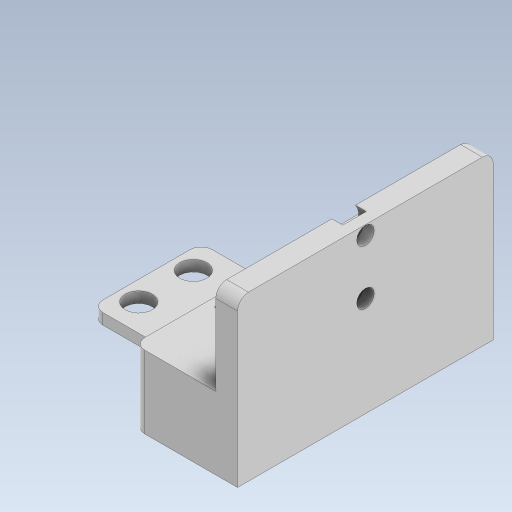
# Autodesk Inventor part: Bracket Servo
Saved by Autodesk Inventor 2023.5 (Build 275446000, 446)
## iProperties
Created: 2025-10-05
Part Number: Bracket Servo
Material: Generic
Document SubType Name: Modeling
Designer: Guntur
Density: 1 g/cm^3
Appearance: Default
Author: Guntur
## iProperties of the stored document Bracket Servo_3DPrint.ipt
Created: 2025-10-05
Part Number: Bracket Servo_3DPrint
Material: Generic
Document SubType Name: Modeling
Designer: Guntur
Density: 1 g/cm^3
Appearance: Default
Author: Guntur
Autodesk Inventor part; units mm, degrees
ref_plane "YZ Plane" through (0, 0, 0) normal (1, 0, 0) x (0, 1, 0)
ref_plane "XZ Plane" through (0, 0, 0) normal (0, 1, 0) x (-1, 0, 0)
ref_plane "XY Plane" through (0, 0, 0) normal (0, 0, 1) x (1, 0, 0)
sketch "Sketch1" plane through (0, 0, 0) normal (0, 1, 0) x (-1, 0, 0)
  line L0 (6, 11.4375) -> (-6, 11.4375)
  line L1 (-6, 11.4375) -> (-6, -11.4375)
  line L2 (-6, -11.4375) -> (6, -11.4375)
  line L3 (6, -11.4375) -> (6, 11.4375)
  line L4 (6, 11.4375) -> (-6, -11.4375) construction
  line L5 (-6, 11.4375) -> (6, -11.4375) construction
  line L6 (6, 16.15) -> (-6, 16.15)
  line L7 (-6, 16.15) -> (-6, -16.15)
  line L8 (-6, -16.15) -> (6, -16.15)
  line L9 (6, -16.15) -> (6, 16.15)
  line L10 (6, 16.15) -> (-6, -16.15) construction
  line L11 (-6, 16.15) -> (6, -16.15) construction
  circle A0 centre (0, -5.4375) radius 2.5
  circle A1 centre (-2.5, 17.225) radius 2.5
  line L12 (7.5, 17.5) -> (-7.5, 17.5)
  line L13 (-7.5, 17.5) -> (-7.5, -17.5)
  line L14 (-7.5, -17.5) -> (7.5, -17.5)
  line L15 (7.5, -17.5) -> (7.5, 17.5)
  line L16 (7.5, 17.5) -> (-7.5, -17.5) construction
  line L17 (-7.5, 17.5) -> (7.5, -17.5) construction
  line L18 (7.5, 17.5) -> (-7.5, 17.5)
  line L19 (-7.5, 17.5) -> (-7.5, 29.3625)
  line L20 (-7.5, 29.3625) -> (7.5, 29.3625)
  line L21 (7.5, 29.3625) -> (7.5, 17.5)
  circle A2 centre (15, 0.9625) radius 2.5
  circle A3 centre (15, 10.9625) radius 2.5
  circle A4 centre (25, 10.9625) radius 2.5
  circle A5 centre (25, 0.9625) radius 2.5
  line L22 (28.6005, 5.9313) -> (28.6005, -4.0687)
  line L23 (28.6005, -4.0687) -> (7.5, -4.0687)
  line L24 (28.6005, 5.9313) -> (28.6005, 15.9313)
  line L25 (28.6005, 15.9313) -> (7.5, 15.9313)
  line L26 (-7.5, -17.5) -> (-11.5, -17.5)
  line L27 (-11.5, -17.5) -> (-11.5, 29.3625)
  line L28 (-11.5, 29.3625) -> (-7.5, 29.3625)
  line L29 (-7.5, 29.3625) -> (-7.5, -17.5)
  point P0 (0, 0)
  point P1 (0, -11.4375)
  point P2 (-0.2429, 16.15)
  point P3 (-4.7571, 16.15)
  point P4 (-4.9848, 17.5)
  point P5 (-0.0152, 17.5)
  dimension "d2" = 12
  dimension "d3" = 22.875
  dimension "d4" = 12
  dimension "d5" = 32.3
  dimension "d6" = 5
  dimension "d7" = 6
  dimension "d8" = 5
  dimension "d9" = 22.8
  dimension "d10" = 15
  dimension "d11" = 35
  dimension "d17" = 5
  dimension "d18" = 15
  dimension "d19" = 6.4
  dimension "d20" = 5
  dimension "d21" = 10
  dimension "d22" = 5
  dimension "d23" = 10
  dimension "d25" = 5
  dimension "d27" = 10
  dimension "d31" = 4
  dimension "d46" = 10
  constraints: 60 end point, 10 parallel, 7 midpoint, 6 centre point, 6 perpendicular, 5 horizontal, 1 point on line
  measures "d2" distance of L2.end L1.end
  measures "d3" distance of L1.end L0.end
  measures "d4" distance of L8.end L7.end
  measures "d5" distance of L7.end L6.end
  measures "d6" diameter of A0
  measures "d7" distance of point (0, -11.438) A0.centre
  measures "d8" diameter of A1
  measures "d9" distance of A1.centre A0.centre
  measures "d10" distance of L14.end L13.end
  measures "d11" distance of L13.end L12.end
  measures "d17" diameter of A2
  measures "d18" horizontal distance of A0.centre A2.centre
  measures "d19" vertical distance of A2.centre A0.centre
  measures "d20" diameter of A3
  measures "d21" distance of A2.centre A3.centre
  measures "d22" diameter of A4
  measures "d23" distance of A3.centre A4.centre
  measures "d25" diameter of A5
  measures "d27" distance of L22.start L22.end
  measures "d31" distance of L27.end L28.end
  measures "d46" distance from line of L21 A1.centre
extrude "Extrusion1" add sketch "Sketch1" along normal blind 10.8 contours L0 L7 L6 A1 L9 | L9 L8 L7 L2
extrude "Extrusion2" add sketch "Sketch1" along normal blind 13.3 contours L9 L6 A1 L12 L15 L14 L13 L7 L1 L8 L3 | L12 L19 L20 L21 A1
extrude "Extrusion3" add sketch "Sketch1" along normal blind 2 contours L25 L24 L22 L23 L15
fillet "Fillet1" radius 2 6 edges at (-7.5, 1, -4.0687) (-7.5, 1, 15.9313) (-28.6005, 1, 15.9313) (-28.6005, 1, -4.0687) (-7.5, 6.65, 29.3625) (-7.5, 6.65, -17.5)
extrude "Extrusion4" add sketch "Sketch1" along normal blind 30 contours L13 L26 L27 L28 L19
sketch "Sketch2" plane through (7.5, 13.3, 29.3625) normal (-1, 0, 0) x (0, 0, 1)
  circle A0 centre (-23.4313, 5) radius 1.6
  circle A1 centre (-23.4313, 5) radius 2.75
  circle A2 centre (-23.4313, 15) radius 1.6
  circle A3 centre (-23.4313, 15) radius 2.75
  line L0 (0, 0) -> (-46.8625, 0) projected
  point P0 (-29.3625, -13.3)
  dimension "d34" = 3.2
  dimension "d35" = 5.5
  dimension "d36" = 3.2
  dimension "d37" = 5.5
  dimension "d39" = 5
  dimension "d40" = 10
  constraints: 4 centre point, 2 coincident
  measures "d34" diameter of A0
  measures "d35" diameter of A1
  measures "d36" diameter of A2
  measures "d37" diameter of A3
  measures "d39" distance from line of L0 A0.centre
  measures "d40" distance of A0.centre A2.centre
extrude "Extrusion5" cut sketch "Sketch2" against normal blind 4 contours A0 | A2
extrude "Extrusion6" cut sketch "Sketch2" against normal blind 2
fillet "Fillet2" radius 2 2 edges at (9.5, 30, 29.3625) (9.5, 30, -17.5)
body "Solid1"
